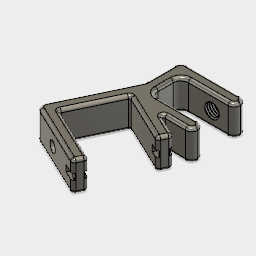
Clamp-Projector (Autodesk Fusion 360 design; units mm, degrees)
Autodesk Fusion 360 part; units mm, degrees
sketch "Sketch1" plane through (0, 0, 0) normal (0, 1, 0) x (1, 0, 0)
  line L0 (-5, 15) -> (30, 15)
  line L1 (30, 15) -> (30, -5)
  line L2 (30, -5) -> (-5, -5)
  line L3 (-5, -5) -> (-5, 15)
  line L4 (30, 23) -> (-13, 23)
  line L5 (-13, 23) -> (-13, -13)
  line L6 (-13, -13) -> (30, -13)
  line L7 (30, -13) -> (30, 23)
  line L8 (-13, -13) -> (-49.000001, -13)
  line L9 (-49.000001, -13) -> (-49.000001, 23)
  line L10 (-49.000001, 23) -> (-13, 23)
  line L11 (-13, 23) -> (-13, -13)
  line L12 (30, -5) -> (25, -5)
  line L13 (25, -5) -> (25, -13)
  line L14 (25, -13) -> (30, -13)
  line L15 (30, -13) -> (30, -5)
  dimension "d7" = 36.000001
  dimension "d21" = 8
  dimension "d22" = 5
  constraint horizontal L0
  constraint vertical L1
  constraint horizontal L2
  constraint vertical L3
  constraint horizontal L4
  constraint vertical L5
  constraint horizontal L6
  constraint vertical L7
  constraint horizontal L8
  constraint vertical L9
  constraint horizontal L10
  constraint vertical L11
  constraint horizontal L12
  constraint vertical L13
  constraint horizontal L14
  constraint vertical L15
  measures "d7" distance of origin
  measures "d21" distance of origin
extrude "Extrude1" add sketch "Sketch1" along normal blind 20 contours L0 L2 L3 L4 L5 L6 L7 L11 L13 | L2 L6 L7 L12 L13 L14 L15 picked at (4, 20.333333) picked at (26.666667, -7.666667)
fillet "Fillet2" radius 5 2 edges at (-5, 10, 5) (-5, 10, -15)
sketch "Sketch2" plane through (0, 0, -15) normal (0, 0, 1) x (1, 0, 0)
  line L0 (0, 20) -> (0, 0)
  line L1 (0, 0) -> (30, 0)
  line L2 (30, 0) -> (30, 20)
  line L3 (30, 20) -> (0, 20)
  circle A0 centre (15, 10) radius 5
extrude "Extrude2" cut sketch "Sketch2" against normal blind 10 contours A0 picked at (15.12455, 11.440906)
thread "Thread1" "ISO Metric profile 10.0 M10x1.5 6H" major diameter 10.198 minor diameter 8.526 pitch 1.5 angle 60 modelled right hand crest width 0.1875 on face at (19.975154, 9.502161, -17.666667) crest through (19.263, 10, -14.15625)
sketch "Sketch5" plane through (0, 0, 0) normal (0, -1, 0) x (1, 0, 0)
  line L0 (30, 5) -> (30, 13)
  line L1 (30, 13) -> (-13, 13)
  line L2 (-13, 13) -> (-13, -23)
  line L3 (-13, -23) -> (30, -23)
  line L4 (30, -23) -> (30, -15)
  line L5 (30, -15) -> (0, -15)
  arc A0 (-5, -10) -> (0, -15) centre (0, -10) ccw
  line L6 (-5, -10) -> (-5, 0)
  arc A1 (0, 5) -> (-5, 0) centre (0, 0) ccw
  line L7 (0, 5) -> (30, 5)
  line L8 (-13, -15) -> (-43, -15)
  line L9 (-43, -15) -> (-43, 15)
  line L10 (-43, 15) -> (-13, 15)
  line L11 (-13, 15) -> (-13, -15)
  line L12 (-13, 15) -> (-35, 15)
  line L13 (-35, 15) -> (-35, -7)
  line L14 (-35, -7) -> (-13, -7)
  line L15 (-13, -7) -> (-13, 15)
  line L16 (-13, 13) -> (17, 13)
  line L17 (17, 13) -> (17, 43)
  line L18 (17, 43) -> (-13, 43)
  line L19 (-13, 43) -> (-13, 13)
  line L20 (17, 13) -> (-5, 13)
  line L21 (-5, 13) -> (-5, 35)
  line L22 (-5, 35) -> (17, 35)
  line L23 (17, 35) -> (17, 13)
  dimension "d10" = 30
  dimension "d11" = 30
  dimension "d12" = 22
  dimension "d13" = 22
  dimension "d14" = 30
  dimension "d15" = 30
  dimension "d16" = 22
  dimension "d17" = 22
  constraint horizontal L8
  constraint vertical L9
  constraint horizontal L10
  constraint vertical L11
  constraint coincident L2 A1.centre
  constraint horizontal L12
  constraint vertical L13
  constraint horizontal L14
  constraint vertical L15
  constraint horizontal L16
  constraint vertical L17
  constraint horizontal L18
  constraint vertical L19
  constraint horizontal L20
  constraint vertical L21
  constraint horizontal L22
  constraint vertical L23
  measures "d12" distance of A1.centre
  measures "d14" distance of A1.centre
  measures "d17" distance of A1.centre
sketch "Sketch8" plane through (0, 20, 0) normal (0, 1, 0) x (-1, 0, 0)
  line L0 (-30, 13) -> (-30, 5)
  line L1 (-30, 5) -> (0, 5)
  arc A0 (5, 0) -> (0, 5) centre (0, 0) ccw
  line L2 (5, 0) -> (5, -10)
  arc A1 (0, -15) -> (5, -10) centre (0, -10) ccw
  line L3 (0, -15) -> (-30, -15)
  line L4 (-30, -15) -> (-30, -23)
  line L5 (-30, -23) -> (13, -23)
  line L6 (13, -23) -> (13, 13)
  line L7 (13, 13) -> (-30, 13)
  line L8 (-30, 13) -> (10, 13)
  line L9 (10, 13) -> (-30, 32)
  line L10 (10, 13) -> (25.016989, 44.614713)
  line L11 (25.016989, 44.614713) -> (-11.114112, 61.776985)
  line L12 (-11.114112, 61.776985) -> (-7.681657, 69.003205)
  line L13 (-7.681657, 69.003205) -> (35.675663, 48.408478)
  line L14 (35.675663, 48.408478) -> (13, 0.670241)
  line L15 (-30, 13) -> (-22.63641, 28.502295)
  line L16 (-22.63641, 28.502295) -> (-26.318205, 20.751148)
  line L17 (-26.318205, 20.751148) -> (-10, 13)
  dimension "d30" = 19
  dimension "d31" = 40
  dimension "d32" = 35
  dimension "d33" = 90
  dimension "d34" = 40
  dimension "d35" = 90
  dimension "d36" = 8
  dimension "d37" = 48
  constraint horizontal L8
  constraint coincident L6 A0.centre
  constraint perpendicular L13 L14
  constraint coincident L9 A0.centre
  constraint perpendicular L9 L15
  constraint midpoint L15 A0.centre
  constraint midpoint L8
  measures "d30" distance of A0.centre
  measures "d33" angle of L9 L10
  measures "d34" distance of A0.centre
  measures "d35" angle of L10 L11
  measures "d36" distance of A0.centre
  measures "d37" distance of A0.centre
extrude "Extrude5" add sketch "Sketch8" against normal blind 20 contours L7 L8 L15 L17 | L7 L8 L9 L15 L16 L17 | L6 L7 L10 L11 L12 L13 L14 picked at (-22.106068, 15.583716) picked at (-7.54547, 18.167432) picked at (17.670331, 54.008799)
sketch "Sketch9" plane through (-21.896132, 0, 46.09712) normal (0.429057, 0, -0.903278) x (-0.903278, 0, -0.429057)
  line L0 (3.455036, 20) -> (-36.544964, 20)
  line L1 (-36.544964, 20) -> (-36.544964, 0)
  line L2 (-36.544964, 0) -> (3.455036, 0)
  line L3 (3.455036, 0) -> (3.455036, 20)
  line L4 (3.455036, 10) -> (-6.544964, 10)
  circle A0 centre (-10.044964, 10) radius 3.5
  dimension "d40" = 10
  dimension "d41" = 7
  constraint midpoint L3 origin
  constraint coincident origin A0
  measures "d41" diameter of A0
extrude "Extrude6" cut sketch "Sketch9" against normal blind 20 contours A0 picked at (-8.993833, 9.818436)
sketch "Sketch10" plane through (-25.328586, 0, 53.32334) normal (-0.429057, 0, 0.903278) x (0.903278, 0, 0.429057)
  circle A0 centre (10.044964, 10) radius 3.5
  line L0 (36.544964, 20) -> (-11.455036, 20)
  line L1 (-11.455036, 20) -> (-11.455036, 0)
  line L2 (-11.455036, 0) -> (36.544964, 0)
  line L3 (36.544964, 0) -> (36.544964, 20)
  line L4 (36.544964, 10) -> (32.544964, 10)
  line L5 (32.544964, 10) -> (32.544964, 12)
  line L6 (32.544964, 12) -> (36.544964, 12)
  line L7 (36.544964, 12) -> (36.544964, 10)
  line L8 (36.544964, 10) -> (32.544964, 10)
  line L9 (32.544964, 10) -> (32.544964, 8)
  line L10 (32.544964, 8) -> (36.544964, 8)
  line L11 (36.544964, 8) -> (36.544964, 10)
  line L12 (32.544964, 12) -> (28.544964, 12)
  line L13 (28.544964, 12) -> (28.544964, 8)
  line L14 (28.544964, 8) -> (32.544964, 8)
  line L15 (32.544964, 8) -> (32.544964, 12)
  dimension "d44" = 2
  dimension "d45" = 4
  dimension "d46" = 4
  dimension "d47" = 2
  dimension "d48" = 4
  constraint horizontal L4
  constraint vertical L5
  constraint horizontal L6
  constraint vertical L7
  constraint midpoint L3 origin
  constraint horizontal L8
  constraint vertical L9
  constraint horizontal L10
  constraint vertical L11
  constraint horizontal L12
  constraint vertical L13
  constraint horizontal L14
  constraint vertical L15
extrude "Extrude7" cut sketch "Sketch10" against normal blind 20 contours L5 L9 L12 L13 L14 L15 picked at (29.878297, 10)
sketch "Sketch11" plane through (-25.328586, 0, 53.32334) normal (-0.429057, 0, 0.903278) x (0.903278, 0, 0.429057)
  line L0 (28.544964, 12) -> (32.544964, 12)
  line L1 (32.544964, 12) -> (32.544964, 8)
  line L2 (32.544964, 8) -> (28.544964, 8)
  line L3 (28.544964, 8) -> (28.544964, 12)
  circle A0 centre (10.044964, 10) radius 3.5
  line L4 (36.544964, 20) -> (-11.455036, 20)
  line L5 (-11.455036, 20) -> (-11.455036, 0)
  line L6 (-11.455036, 0) -> (36.544964, 0)
  line L7 (36.544964, 0) -> (36.544964, 20)
  line L8 (32.544964, 12) -> (36.544964, 12)
  line L9 (36.544964, 12) -> (36.544964, 8)
  line L10 (36.544964, 8) -> (32.544964, 8)
  line L11 (32.544964, 8) -> (32.544964, 12)
  dimension "d51" = 4
  dimension "d52" = 4
  constraint horizontal L8
  constraint vertical L9
  constraint horizontal L10
  constraint vertical L11
  measures "d51" distance of origin
  measures "d52" distance of origin
extrude "Extrude8" cut sketch "Sketch11" against normal blind 1.5 contours L1 L7 L8 L9 L10 L11 picked at (35.21163, 9.333333)
sketch "Sketch12" plane through (-21.896132, 0, 46.09712) normal (0.429057, 0, -0.903278) x (-0.903278, 0, -0.429057)
  line L0 (-32.544964, 12) -> (-28.544964, 12)
  line L1 (-28.544964, 12) -> (-28.544964, 8)
  line L2 (-28.544964, 8) -> (-32.544964, 8)
  line L3 (-32.544964, 8) -> (-32.544964, 12)
  circle A0 centre (-10.044964, 10) radius 3.5
  line L4 (3.455036, 20) -> (-36.544964, 20)
  line L5 (-36.544964, 20) -> (-36.544964, 0)
  line L6 (-36.544964, 0) -> (3.455036, 0)
  line L7 (3.455036, 0) -> (3.455036, 20)
  line L8 (-32.544964, 12) -> (-36.544964, 12)
  line L9 (-36.544964, 12) -> (-36.544964, 8)
  line L10 (-36.544964, 8) -> (-32.544964, 8)
  line L11 (-32.544964, 8) -> (-32.544964, 12)
  dimension "d55" = 4
  dimension "d56" = 4
  constraint horizontal L8
  constraint vertical L9
  constraint horizontal L10
  constraint vertical L11
extrude "Extrude9" cut sketch "Sketch12" against normal blind 1.5 contours L3 L5 L8 L9 L10 L11 picked at (-35.21163, 9.333333)
sketch "Sketch13" plane through (0, 20, 0) normal (0, 1, 0) x (-1, 0, 0)
  line L0 (-30, 13) -> (-30, 5)
  line L1 (-30, 5) -> (0, 5)
  arc A0 (5, 0) -> (0, 5) centre (0, 0) ccw
  line L2 (5, 0) -> (5, -10)
  arc A1 (0, -15) -> (5, -10) centre (0, -10) ccw
  line L3 (0, -15) -> (-30, -15)
  line L4 (-30, -15) -> (-30, -23)
  line L5 (-30, -23) -> (13, -23)
  line L6 (13, -23) -> (13, 0.670241)
  line L7 (13, 0.670241) -> (35.675663, 48.408478)
  line L8 (35.675663, 48.408478) -> (-7.681657, 69.003205)
  line L9 (-7.681657, 69.003205) -> (-11.114112, 61.776985)
  line L10 (-11.114112, 61.776985) -> (25.016989, 44.614713)
  line L11 (25.016989, 44.614713) -> (10, 13)
  line L12 (10, 13) -> (-22.63641, 28.502295)
  line L13 (-22.63641, 28.502295) -> (-30, 13)
  line L14 (-22.63641, 28.502295) -> (-26.068865, 21.276075)
  line L15 (-26.068865, 21.276075) -> (-8.003314, 12.694939)
  line L16 (-8.003314, 12.694939) -> (-30, 13)
  dimension "d59" = 8
  dimension "d60" = 20
  constraint coincident A0.centre origin
  measures "d59" distance of A0.centre
extrude "Extrude10" cut sketch "Sketch13" against normal blind 20 contours L13 L15 L16 picked at (-21.357393, 15.657005)
sketch "Sketch14" plane through (-6.879143, 0, 14.482407) normal (-0.429057, 0, 0.903278) x (0.903278, 0, 0.429057)
  line L0 (32.676064, 20) -> (-3.455036, 20)
  line L1 (-3.455036, 20) -> (-3.455036, 0)
  line L2 (-3.455036, 0) -> (32.676064, 0)
  line L3 (32.676064, 0) -> (32.676064, 20)
  line L4 (32.676064, 10) -> (30.676064, 10)
  line L5 (30.676064, 10) -> (30.676064, 8)
  line L6 (30.676064, 8) -> (32.676064, 8)
  line L7 (32.676064, 8) -> (32.676064, 10)
  line L8 (30.676064, 8) -> (26.676064, 8)
  line L9 (26.676064, 8) -> (26.676064, 12)
  line L10 (26.676064, 12) -> (30.676064, 12)
  line L11 (30.676064, 12) -> (30.676064, 8)
  dimension "d63" = 2
  dimension "d64" = 2
  dimension "d65" = 4
  dimension "d66" = 4
  constraint horizontal L4
  constraint vertical L5
  constraint horizontal L6
  constraint vertical L7
  constraint midpoint L3 origin
  constraint horizontal L8
  constraint vertical L9
  constraint horizontal L10
  constraint vertical L11
  measures "d66" distance of origin
extrude "Extrude11" cut sketch "Sketch14" against normal blind 8 contours L5 L8 L9 L10 L11 picked at (28.009397, 10)
sketch "Sketch15" plane through (-6.879143, 0, 14.482407) normal (-0.429057, 0, 0.903278) x (0.903278, 0, 0.429057)
  line L0 (26.676064, 8) -> (26.676064, 12)
  line L1 (26.676064, 12) -> (30.676064, 12)
  line L2 (30.676064, 12) -> (30.676064, 8)
  line L3 (30.676064, 8) -> (26.676064, 8)
  line L4 (32.676064, 20) -> (-3.455036, 20)
  line L5 (-3.455036, 20) -> (-3.455036, 0)
  line L6 (-3.455036, 0) -> (32.676064, 0)
  line L7 (32.676064, 0) -> (32.676064, 20)
  line L8 (30.676064, 12) -> (32.676064, 12)
  line L9 (32.676064, 12) -> (32.676064, 8)
  line L10 (32.676064, 8) -> (30.676064, 8)
  line L11 (30.676064, 8) -> (30.676064, 12)
  dimension "d69" = 4
  dimension "d70" = 2
  constraint horizontal L8
  constraint vertical L9
  constraint horizontal L10
  constraint vertical L11
extrude "Extrude12" cut sketch "Sketch15" against normal blind 1.5 contours L2 L7 L8 L9 L10 L11 picked at (31.34273, 9.333333)
fillet "Fillet8" radius 5 1 edges at (-13, 10, 0.670241)
sketch "Sketch16" plane through (-3.446689, 0, 7.256187) normal (0.429057, 0, -0.903278) x (-0.903278, 0, -0.429057)
  line L0 (-26.676064, 12) -> (-26.676064, 8)
  line L1 (-26.676064, 8) -> (-30.676064, 8)
  line L2 (-30.676064, 8) -> (-30.676064, 12)
  line L3 (-30.676064, 12) -> (-26.676064, 12)
  line L4 (-12.676064, 20) -> (-32.676064, 20)
  line L5 (-32.676064, 20) -> (-32.676064, 0)
  line L6 (-32.676064, 0) -> (-12.676064, 0)
  line L7 (-12.676064, 0) -> (-12.676064, 20)
  line L8 (-30.676064, 12) -> (-32.676064, 12)
  line L9 (-32.676064, 12) -> (-32.676064, 8)
  line L10 (-32.676064, 8) -> (-30.676064, 8)
  line L11 (-30.676064, 8) -> (-30.676064, 12)
  dimension "d74" = 4
  dimension "d75" = 2
  constraint horizontal L8
  constraint vertical L9
  constraint horizontal L10
  constraint vertical L11
extrude "Extrude13" cut sketch "Sketch16" against normal blind 1.5 contours L2 L5 L8 L9 L10 L11 picked at (-32.009397, 9.333333)
fillet "Fillet9" radius 4 3 edges at (30, 10, -15) (30, 10, -23) (-13, 10, -23)
fillet "Fillet10" radius 4 1 edges at (-35.675663, 10, 48.408478)
fillet "Fillet11" radius 4 1 edges at (30, 10, 5)
fillet "Fillet12" radius 4 1 edges at (30, 10, 13)
fillet "Fillet13" radius 2 8 edges at (7.681657, 16, 69.003205) (11.114112, 16, 61.776985) (7.681657, 4, 69.003205) (11.114112, 4, 61.776985) (22.63641, 16, 28.502295) (22.63641, 4, 28.502295) (26.068865, 16, 21.276075) (26.068865, 4, 21.276075)
fillet "Fillet14" radius 1 2 edges at (-25.016989, 10, 44.614713) (-10, 10, 13)
fillet "Fillet15" radius 1 1 edges at (8.003314, 10, 12.694939)
fillet "Fillet16" radius 1 4 edges at (4.712132, 10, 65.932062) (6.857416, 10, 61.415674) (21.47344, 10, 26.289265) (23.618724, 10, 21.772878)
fillet "Fillet17" radius 2 30 edges at (28.789185, 20, 11.811658) (19.26584, 20, 12.851133) (11.59892, 20, 13.531737) (18.203072, 20, 17.539823) (25.288401, 20, 21.553867) (24.352637, 20, 24.889185) (22.358618, 20, 27.721832) (5.866566, 20, 20.536619) (-9.861104, 20, 13.390232) (-17.508494, 20, 28.807357) (-24.626757, 20, 44.475817) (-7.403077, 20, 52.981321) (10.333648, 20, 62.054777) (9.397884, 20, 65.390095) (7.403865, 20, 68.222742) (-13.093725, 20, 59.134899) (-34.114736, 20, 47.852894) (-23.721524, 20, 23.24187) (-13.122402, 20, 0.642648) (-13, 20, -9.728456) (-11.828427, 20, -21.828427) (8.5, 20, -23) (28.828427, 20, -21.828427) (28.828427, 20, -16.171573) (13, 20, -15) (-3.535534, 20, -13.535534) (-5, 20, -5) (-3.535534, 20, 3.535534) (13, 20, 5) (28.828427, 20, 6.171573)
fillet "Fillet18" radius 2 30 edges at (28.828427, 0, 6.171573) (28.789185, 0, 11.811658) (19.26584, 0, 12.851133) (11.59892, 0, 13.531737) (18.203072, 0, 17.539823) (25.288401, 0, 21.553867) (24.352637, 0, 24.889185) (22.358618, 0, 27.721832) (5.866566, 0, 20.536619) (-9.861104, 0, 13.390232) (-17.508494, 0, 28.807357) (-24.626757, 0, 44.475817) (-7.403077, 0, 52.981321) (10.333648, 0, 62.054777) (9.397884, 0, 65.390095) (7.403865, 0, 68.222742) (-13.093725, 0, 59.134899) (-34.114736, 0, 47.852894) (-23.721524, 0, 23.24187) (-13.122402, 0, 0.642648) (-13, 0, -9.728456) (-11.828427, 0, -21.828427) (8.5, 0, -23) (28.828427, 0, -21.828427) (28.828427, 0, -16.171573) (13, 0, -15) (-3.535534, 0, -13.535534) (-5, 0, -5) (-3.535534, 0, 3.535534) (13, 0, 5)
